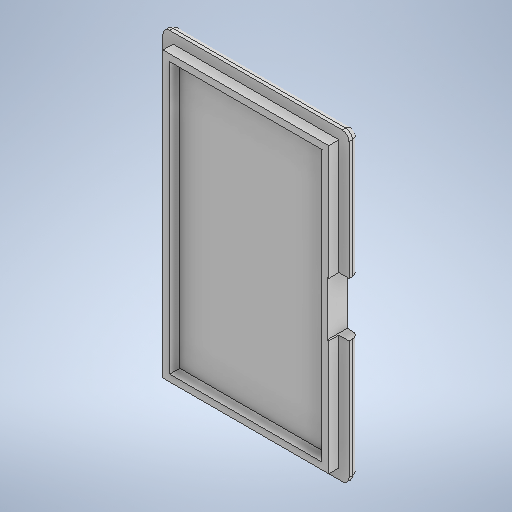
# Autodesk Inventor part: adapter_box_lid
Saved by Autodesk Inventor 2025 (Build 290162000, 162)
## iProperties
Created: 2025-02-26
Part Number: adapter_box_lid
Material: Všeobecné
Document SubType Name: Modeling
Designer: lukas
Density: 1 g/cm^3
Appearance: Výchozí
Author: lukas
## iProperties of the stored document adapter_box_lid_3D tisk.ipt
Created: 2025-02-26
Part Number: adapter_box_lid_3D tisk
Material: Všeobecné
Document SubType Name: Modeling
Designer: lukas
Density: 1 g/cm^3
Appearance: Výchozí
Author: lukas
Autodesk Inventor part; units mm, degrees
ref_plane "YZ Plane" through (0, 0, 0) normal (1, 0, 0) x (0, 1, 0)
ref_plane "XZ Plane" through (0, 0, 0) normal (0, 1, 0) x (-1, 0, 0)
ref_plane "XY Plane" through (0, 0, 0) normal (0, 0, 1) x (1, 0, 0)
sketch "Náčrt1" plane through (0, 0, 0) normal (0, 0, 1) x (1, 0, 0)
  line L0 (0, 63) -> (0, -63) projected
  line L1 (-38.5, 0) -> (38.5, 0) projected
  line L2 (27.5, -45) -> (-27.5, -45)
  line L3 (-27.5, -45) -> (-27.5, 45)
  line L4 (-27.5, 45) -> (27.5, 45)
  line L5 (27.5, 45) -> (27.5, -45)
  point P0 (0, 0)
  dimension "d0" = 55
  dimension "d1" = 90
  constraints: 8 end point, 2 parallel, 1 horizontal, 1 perpendicular, 2 other
  measures "d0" distance of L3.end L4.end
  measures "d1" distance of L4.end L2.start
extrude "Vysunutí1" add sketch "Náčrt1" along normal blind 3
sketch "Náčrt2" plane through (0, 0, 3) normal (0, 0, 1) x (1, 0, 0)
  line L0 (27.5, 45) -> (-27.5, 45) projected
  line L1 (-27.5, 45) -> (-27.5, -45) projected
  line L2 (-27.5, -45) -> (27.5, -45) projected
  line L3 (27.5, -45) -> (27.5, 45) projected
  line L4 (-27.5, 45) -> (-27.5, -45) projected
  line L5 (0, 63) -> (0, -63) projected
  line L6 (-38.5, 0) -> (38.5, 0) projected
  line L7 (24.5, -42) -> (-24.5, -42)
  line L8 (-24.5, -42) -> (-24.5, 42)
  line L9 (-24.5, 42) -> (24.5, 42)
  line L10 (24.5, 42) -> (24.5, -42)
  line L11 (-22.5, 40) -> (-22.5, -40)
  line L12 (-22.5, -40) -> (22.5, -40)
  line L13 (22.5, -40) -> (22.5, 40)
  line L14 (22.5, 40) -> (-22.5, 40)
  line L15 (-22.5, 0) -> (-24.5, 0)
  line L16 (-24.5, 0) -> (-24.5, -42)
  line L17 (-24.5, -42) -> (-22.5, -42)
  line L18 (-22.5, -42) -> (-22.5, 0)
  line L19 (22.5, 0) -> (24.5, 0)
  line L20 (24.5, 0) -> (24.5, -42)
  line L21 (24.5, -42) -> (22.5, -42)
  line L22 (22.5, -42) -> (22.5, 0)
  line L23 (24.5, -42) -> (-22.5, -42)
  line L24 (-22.5, -42) -> (-22.5, -40)
  line L25 (-22.5, -40) -> (24.5, -40)
  line L26 (24.5, -40) -> (24.5, -42)
  line L27 (-24.5, -42) -> (-22.5, -42)
  line L28 (-22.5, -42) -> (-22.5, -40)
  line L29 (-22.5, -40) -> (-24.5, -40)
  line L30 (-24.5, -40) -> (-24.5, -42)
  point P0 (0, 0)
  point P1 (24.5, 0)
  dimension "d8" = 49
  dimension "d9" = 84
  dimension "d10" = 2
  constraints: 48 end point, 12 parallel, 6 perpendicular, 5 horizontal, 2 midpoint, 5 other
  measures "d8" distance of L8.end L9.end
  measures "d9" distance between parallel lines of L7 L9
  measures "d10" distance between parallel lines of L8 L11
extrude "Vysunutí2" add sketch "Náčrt2" along normal blind 3 contours L9 L10 L6 L13 L14 L5 | L5 L14 L11 L6 L8 L9 | L10 L25 L13 L6 | L10 L7 L22 L25 | L6 L11 L29 L8 | L7 L18 L12 L5 | L5 L12 L22 L7 | L29 L18 L7 L8
sketch "Náčrt3" plane through (0, 0, 0) normal (0, 0, -1) x (-1, 0, 0)
  line L0 (-27.5, 45) -> (27.5, 45) projected
  line L1 (-27.5, -45) -> (-27.5, 45) projected
  line L2 (27.5, -45) -> (-27.5, -45) projected
  line L3 (27.5, 45) -> (27.5, -45) projected
  line L4 (-27.5, -8) -> (-24, -8)
  line L5 (-24, -8) -> (-24, 8)
  line L6 (-24, 8) -> (-27.5, 8)
  line L7 (-27.5, 8) -> (-27.5, -8)
  line L8 (0, -63) -> (0, 63) projected
  line L9 (-38.5, 0) -> (38.5, 0) projected
  point P0 (0, 0)
  point P1 (-27.5, 8)
  dimension "d13" = 3.5
  dimension "d14" = 16
  constraints: 8 end point, 2 parallel, 1 horizontal, 1 perpendicular, 1 point on line, 1 other
  measures "d13" distance of L5.end L6.end
  measures "d14" distance of L4.end L5.end
extrude "Vysunutí3" cut sketch "Náčrt3" against normal through all contours L6 L5 L9 L1 | L9 L5 L4 L1
fillet "Zaoblení1" radius 2 9 edges at (27.5, 26.5, 0) (0, 45, 0) (27.5, 45, 1.5) (-27.5, 45, 1.5) (-27.5, 0, 0) (27.5, -26.5, 0) (0, -45, 0) (27.5, -45, 1.5) (-27.5, -45, 1.5)
